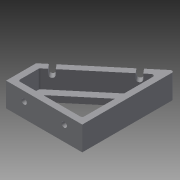
# Autodesk Inventor part: lcd_halterung_162C_rechts
Saved by Autodesk Inventor 2015 (Build 190159000, 159)
## iProperties
Created: 2014-11-18
Part Number: lcd_halterung_162C_rechts
Material: Generisch
Document SubType Name: Modeling
Designer: Zephram
Density: 1 g/cm^3
Appearance: Vorgabe
Author: Zephram
Autodesk Inventor part; units mm, degrees
ref_plane "YZ Plane" through (0, 0, 0) normal (1, 0, 0) x (0, 1, 0)
ref_plane "XZ Plane" through (0, 0, 0) normal (0, 1, 0) x (-1, 0, 0)
ref_plane "XY Plane" through (0, 0, 0) normal (0, 0, 1) x (1, 0, 0)
sketch "Skizze1" plane through (0, 0, 0) normal (0, 0, 1) x (1, 0, 0)
  line L0 (0, 0) -> (0, 46.8858)
  line L1 (0, 46.8858) -> (-38, 15)
  line L2 (-38, 15) -> (-38, 0)
  line L3 (-38, 0) -> (0, 0)
  line L4 (-6.5, 6.5) -> (-6.5, 32.9465)
  line L5 (-6.5, 32.9465) -> (-31.5, 11.969)
  line L6 (-31.5, 11.969) -> (-31.5, 6.5)
  line L7 (-31.5, 6.5) -> (-6.5, 6.5)
  dimension "d0" = 130
  dimension "d1" = 15
  dimension "d2" = 38
  dimension "d3" = 6.5
  dimension "d4" = 6.5
  dimension "d6" = 6.5
  dimension "d7" = 6.5
  constraints: 16 end point, 4 parallel, 2 vertical, 1 perpendicular
  measures "d0" angle of L2 L1
  measures "d1" distance of L2.end L1.end
  measures "d2" distance between parallel lines of L0 L2
  measures "d3" distance between parallel lines of L3 L7
  measures "d4" distance between parallel lines of L0 L4
  measures "d6" distance between parallel lines of L2 L6
  measures "d7" distance between parallel lines of L5 L1
extrude "Extrusion1" add sketch "Skizze1" along normal blind 12
sketch "Skizze2" plane through (0, 0, 12) normal (0, 0, 1) x (1, 0, 0)
  line L0 (-3, 40.4523) -> (-3, 3)
  line L1 (-3, 3) -> (-35, 3)
  line L2 (-35, 3) -> (-35, 13.6011)
  line L3 (-35, 13.6011) -> (-3, 40.4523)
  line L4 (-38, 0) -> (0, 0) projected
  line L5 (-38, 15) -> (-38, 0) projected
  line L6 (0, 46.8858) -> (-38, 15) projected
  line L7 (0, 0) -> (0, 46.8858) projected
  dimension "d10" = 3
  dimension "d11" = 3
  dimension "d12" = 3
  dimension "d13" = 3
  constraints: 8 end point, 4 parallel, 1 vertical
  measures "d10" distance between parallel lines of L5 L2
  measures "d11" distance between parallel lines of L7 L0
  measures "d12" distance between parallel lines of L4 L1
  measures "d13" distance between parallel lines of L6 L3
extrude "Extrusion2" cut sketch "Skizze2" against normal blind 9 contours L0 L1 L2 L3
sketch "Skizze3" plane through (-35, 3, 12) normal (0, 1, 0) x (1, 0, 0)
  line L0 (35, 12) -> (35, 0) projected
  line L1 (35, 0) -> (32, 0) projected
  line L2 (32, 0) -> (32, 9) projected
  line L3 (32, 9) -> (0, 9) projected
  line L4 (0, 9) -> (0, 0) projected
  line L5 (0, 0) -> (-3, 0) projected
  line L6 (-3, 0) -> (-3, 12) projected
  line L7 (-3, 12) -> (35, 12) projected
  line L8 (32, 0) -> (0, 0) projected
  line L9 (0, 4.5) -> (32, 4.5)
  point P0 (6, 4.5)
  point P1 (26, 4.5)
  dimension "d17" = 6
  dimension "d18" = 6
  constraints: 2 end point, 2 midpoint, 2 point on line
  measures "d17" distance from line of L4 point (6, 4.5)
  measures "d18" distance from line of L2 point (26, 4.5)
hole "Bohrung1" at (-29, 3, 7.5) at (-9, 3, 7.5) direction (0, -1, 0) diameter 2.7 depth 8 tip angle 118
fillet "Rundung2" radius 1 9 edges at (0, 46.8858, 6) (-6.5, 32.9465, 1.5) (-3, 40.4523, 7.5) (-31.5, 6.5, 1.5) (-35, 3, 7.5) (-35, 13.6011, 7.5) (-31.5, 11.969, 1.5) (-3, 3, 7.5) (-6.5, 6.5, 1.5)
sketch "Skizze4" plane through (-34.6428, 13.9008, 3) normal (0.6427876, -0.7660444, 0) x (0.7660444, 0.6427876, 0)
  line L0 (45.2229, -3) -> (-4.3825, -3) projected
  line L1 (-4.3825, -3) -> (-4.3825, 9) projected
  line L2 (-4.3825, 9) -> (0, 9) projected
  line L3 (0, 0) -> (0, 9) projected
  line L4 (0, 0) -> (39.1622, 0) projected
  line L5 (39.1622, 0) -> (39.1622, 9) projected
  line L6 (0, 9) -> (39.1622, 9) projected
  line L7 (45.2229, 9) -> (45.2229, -3) projected
  line L8 (39.1622, 9) -> (45.2229, 9) projected
  point P0 (17.6026, -3)
  point P1 (4, 6.5)
  point P2 (35, 6.5)
  dimension "d27" = 2.5
  dimension "d28" = 4
  dimension "d29" = 2.5
  dimension "d30" = 35
  dimension "d31" = 4.1622
  measures "d27" distance from line of L6 point (4, 6.5)
  measures "d28" distance from line of L3 point (4, 6.5)
  measures "d29" distance from line of L6 point (35, 6.5)
  measures "d30" distance from line of L3 point (35, 6.5)
  measures "d31" distance from line of L5 point (35, 6.5)
hole "Bohrung2" at (-31.5786, 16.472, 9.5) at (-7.8312, 36.3984, 9.5) direction (-0.6427876, 0.7660444, 0) diameter 2.7 depth 8 tip angle 118
sketch "Skizze7" plane through (-38, 15, 12) normal (-0.6427876, 0.7660444, 0) x (0.7660444, 0.6427876, 0)
  circle A0 centre (36.8652, 2.5) radius 1.35 projected
  line L0 (38.2152, 2.5) -> (38.2152, 0)
  line L1 (1.8652, 0) -> (41.0274, 0) projected
  line L2 (35.5152, 0) -> (35.5152, 2.5)
  point P0 (19.4679, 12)
  constraints: 4 end point, 2 point on circle, 2 point on line, 2 tangent, 1 vertical
extrude "Extrusion3" cut sketch "Skizze7" against normal blind 6.25 contours L0 L1 L2 A0
sketch "Skizze8" plane through (-38, 15, 12) normal (-0.6427876, 0.7660444, 0) x (0.7660444, 0.6427876, 0)
  circle A0 centre (5.8652, 2.5) radius 1.35 projected
  line L0 (7.2152, 2.5) -> (7.2152, 0)
  line L1 (-9.6418, 0) -> (19.4679, 0) projected
  line L2 (4.5152, 2.5) -> (4.5152, 0)
  point P0 (19.4679, 12)
  constraints: 4 end point, 2 point on circle, 2 point on line, 2 tangent, 1 parallel, 1 vertical
extrude "Extrusion4" cut sketch "Skizze8" against normal blind 6.5 contours L0 L1 L2 A0
